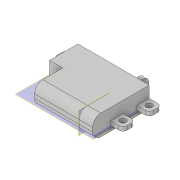
# Autodesk Inventor part: 00_z-slider_chinese_OPPO
Saved by Autodesk Inventor 2019.4 (Build 234330000, 330)
## iProperties
Created: 2021-02-01
Part Number: 00_z-slider_chinese_OPPO
Material: Generic
Document SubType Name: Modeling
Designer: diederichbenedict
Density: 1 g/cm^3
Appearance: Default
Author: diederichbenedict
Autodesk Inventor part; units mm, degrees
ref_plane "YZ Plane" through (0, 0, 0) normal (1, 0, 0) x (0, 1, 0)
ref_plane "XZ Plane" through (0, 0, 0) normal (0, 1, 0) x (-1, 0, 0)
ref_plane "XY Plane" through (0, 0, 0) normal (0, 0, 1) x (1, 0, 0)
sketch "Sketch1" plane through (0, 0, 0) normal (0, 1, 0) x (-1, 0, 0)
  line L0 (0, 0) -> (17.36, 0)
  line L1 (17.36, 0) -> (17.36, 6.9)
  line L2 (17.36, 6.9) -> (0, 6.9)
  line L3 (0, 6.9) -> (0, 0)
  line L4 (0, 6.9) -> (14.12, 6.9)
  line L5 (14.12, 6.9) -> (14.12, 13.8)
  line L6 (14.12, 13.8) -> (0, 13.8)
  line L7 (0, 13.8) -> (0, 6.9)
  dimension "d0" = 17.36
  dimension "d1" = 6.9
  dimension "d2" = 14.12
  dimension "d3" = 6.9
  constraints: 16 end point, 4 parallel, 2 horizontal, 2 perpendicular
  measures "d0" distance of L2.end L1.end
  measures "d1" distance of L1.end L0.end
  measures "d2" distance of L6.end L5.end
  measures "d3" distance of L5.end L4.end
extrude "Extrusion1" add sketch "Sketch1" along normal blind 5
ref_plane "Work Plane1" through (0, 1.2, 0) normal (0, -1, 0) x (1, 0, 0)
sketch "Sketch2" plane through (0, 1.2, 0) normal (0, -1, 0) x (1, 0, 0)
  line L0 (0, 13.8) -> (0, 0) projected
  line L1 (0, 0) -> (-17.36, 0) projected
  line L2 (-17.36, 0) -> (-17.36, 6.9) projected
  line L3 (-17.36, 6.9) -> (-14.12, 6.9) projected
  line L4 (-14.12, 6.9) -> (-14.12, 13.8) projected
  line L5 (-14.12, 13.8) -> (0, 13.8) projected
  line L6 (0, 0) -> (3, 0)
  line L7 (3, 0) -> (3, 3)
  line L8 (3, 3) -> (0, 3)
  line L9 (0, 3) -> (0, 0)
  line L10 (0, 13.8) -> (0, 0) projected
  line L11 (0, 6.4036) -> (3, 6.4036)
  line L12 (3, 6.4036) -> (3, 9.4036)
  line L13 (3, 9.4036) -> (0, 9.4036)
  line L14 (0, 9.4036) -> (0, 6.4036)
  circle A0 centre (1.5, 1.5) radius 0.75
  circle A1 centre (1.5, 7.9036) radius 0.75
  line L15 (-17.36, 0) -> (-17.36, 6.9) projected
  line L16 (-17.36, 0) -> (-20.36, 0)
  line L17 (-20.36, 0) -> (-20.36, 3)
  line L18 (-20.36, 3) -> (-17.36, 3)
  line L19 (-17.36, 3) -> (-17.36, 0)
  circle A2 centre (-18.86, 1.5) radius 0.75
  dimension "d7" = 3
  dimension "d8" = 3
  dimension "d9" = 3
  dimension "d10" = 3
  dimension "d11" = 1.5
  dimension "d12" = 1.5
  dimension "d13" = 3
  dimension "d14" = 3
  dimension "d15" = 1.5
  dimension "d16" = 20.36
  constraints: 24 end point, 6 parallel, 3 centre point, 3 horizontal, 3 perpendicular, 1 point on line
  measures "d7" distance of L8.end L7.end
  measures "d8" distance of L7.end L6.end
  measures "d9" distance of L13.end L12.end
  measures "d10" distance of L12.end L11.end
  measures "d11" diameter of A0
  measures "d12" diameter of A1
  measures "d13" distance of L17.end L18.end
  measures "d14" distance of L16.end L17.end
  measures "d15" diameter of A2
  measures "d16" distance of A2.centre A0.centre
extrude "Extrusion2" add sketch "Sketch2" against normal blind 1 contours L13 L12 L11 L0 | L8 L7 L6 L0 | L2 L16 L17 L18
fillet "Fillet1" radius 1 6 edges at (-20.36, 1.7, 0) (3, 1.7, 9.4036) (3, 1.7, 6.4036) (3, 1.7, 3) (3, 1.7, 0) (-20.36, 1.7, 3)
ref_plane "Work Plane2" through (-3.12, 0, 6.9) normal (-1, 0, 0) x (0, 0, 1)
sketch "Sketch3" plane through (-3.12, 0, 6.9) normal (-1, 0, 0) x (0, 0, 1)
  line L0 (-3.9, 1.2) -> (-6.9, 1.2) projected
  line L1 (-6.9, 0) -> (-6.9, 1.2) projected
  line L2 (-6.9, 0) -> (0, 0) projected
  line L3 (0, 0) -> (0, 5) projected
  line L4 (-6.9, 5) -> (0, 5) projected
  line L5 (-6.9, 2.2) -> (-6.9, 5) projected
  line L6 (-6.9, 2.2) -> (-3.9, 2.2) projected
  line L7 (-3.9, 2.2) -> (-3.9, 1.2) projected
  circle A0 centre (-8.4, 2.5) radius 0.75
  circle A1 centre (-8.4, 2.5) radius 1.5
  line L8 (-6.9, 2.2) -> (-6.9, 5) projected
  dimension "d21" = 1.5
  dimension "d22" = 3
  constraints: 2 centre point, 1 coincident, 1 tangent
  measures "d21" diameter of A0
  measures "d22" diameter of A1
extrude "Extrusion3" add sketch "Sketch3" along normal blind 1 contours A1
fillet "Fillet2" radius 2 2 edges at (-7.06, 5, 13.8) (-7.06, 0, 13.8)
body "Solid1"
